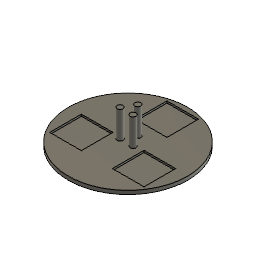
base (Autodesk Fusion 360 design; units mm, degrees)
Autodesk Fusion 360 part; units mm, degrees
note: some values were not read from the file. Set by a fixed rule: which sketch regions a step uses.
sketch "Sketch1" plane through (0, 0, 0) normal (0, 1, 0) x (1, 0, 0)
  line L0 (0, -25) -> (-12.5, -25)
  line L1 (-12.5, -25) -> (12.5, -25)
  line L2 (12.5, -25) -> (37.9, -25)
  circle A0 centre (0, 0) radius 48
  line L3 (37.9, -25) -> (12.5, -25)
  line L4 (12.5, -25) -> (12.5, 0.4)
  line L5 (12.5, 0.4) -> (37.9, 0.4)
  line L6 (37.9, 0.4) -> (37.9, -25)
  line L7 (-12.5, -25) -> (-37.9, -25)
  line L8 (-37.9, -25) -> (-37.9, 0.4)
  line L9 (-37.9, 0.4) -> (-12.5, 0.4)
  line L10 (-12.5, 0.4) -> (-12.5, -25)
  line L11 (-25.2, 0.4) -> (-25.2, -12.3)
  line L12 (12.5, 0.4) -> (25.2, 0.4)
  line L13 (25.2, 0.4) -> (25.2, -12.3)
  line L14 (-25.2, -12.3) -> (25.2, -12.3)
  line L15 (0, -12.3) -> (0, 31.347)
  line L16 (0, 31.347) -> (-25.2, -12.3)
  line L17 (25.2, -12.3) -> (0, 31.347)
  line L18 (0, 31.347) -> (0, 18.647)
  line L19 (0, 18.647) -> (12.7, 18.647)
  line L20 (12.7, 18.647) -> (-12.7, 18.647)
  line L21 (-12.7, 18.647) -> (-12.7, 44.047)
  line L22 (-12.7, 44.047) -> (12.7, 44.047)
  line L23 (12.7, 44.047) -> (12.7, 18.647)
  dimension "d2" = 12.5
  dimension "d3" = 25
  dimension "d4" = 25.4
  dimension "d5" = 96
  dimension "d6" = 25.4
  dimension "d7" = 25.4
  dimension "d8" = 25.4
  dimension "d9" = 25.4
  dimension "d10" = 12.7
  dimension "d11" = 12.7
  dimension "d12" = 12.7
  dimension "d13" = 43.647
  dimension "d14" = 12.7
  dimension "d15" = 12.7
  dimension "d16" = 25.4
  dimension "d17" = 25.4
  constraint horizontal L0
  constraint parallel L0 L1
  constraint parallel L1 L2
  constraint coincident A0.centre origin
  constraint horizontal L3
  constraint vertical L4
  constraint horizontal L5
  constraint vertical L6
  constraint horizontal L7
  constraint vertical L8
  constraint horizontal L9
  constraint vertical L10
  constraint midpoint L9 L11.start
  constraint perpendicular L9 L11
  constraint perpendicular L4 L12
  constraint perpendicular L12 L13
  constraint midpoint L14 L15.start
  constraint perpendicular L14 L15
  constraint parallel L15 L18
  constraint perpendicular L18 L19
  constraint horizontal L20
  constraint vertical L21
  constraint horizontal L22
  constraint vertical L23
  measures "d2" distance of L0.start L0.end
  measures "d3" distance of L0.end L1.end
  measures "d4" distance of L1.end L2.end
  measures "d5" diameter of A0
  measures "d6" distance of L2.end L1.end
  measures "d7" distance of L2.end L5.end
  measures "d8" distance of L0.end L7.end
  measures "d9" distance of L0.end L9.end
  measures "d10" distance of L11.start L11.end
  measures "d11" distance of L4.end L12.end
  measures "d12" distance of L12.end L13.end
  measures "d13" distance of L15.start L15.end
  measures "d14" distance of L15.end L18.end
  measures "d15" distance of L18.end L19.end
  measures "d16" distance of L19.end L20.end
  measures "d17" distance of L19.end L22.end
extrude "Extrude1" add sketch "Sketch1" along normal blind 3 contours L0 L1 L4 L10 L14 | L9 L10 L14 L15 L16 L20 | L4 L5 L12 L14 L15 L17 L19 L20 | A0
extrude "Extrude2" add sketch "Sketch1" along normal blind 1.5 contours L7 L8 L9 L10 L11 L14 | L2 L3 L4 L5 L6 L13 L14 | L9 L10 L14 L16 | L4 L5 L12 L14 L17 | L9 L11 L16 | L5 L12 L13 L17 | L15 L16 L18 L20 | L15 L17 L18 L19 L20 | L16 L17 L19 L20 L21 L22 L23
sketch "Sketch2" plane through (0, 3, 0) normal (0, 1, 0) x (-1, 0, 0)
  line L0 (-12.5, 25) -> (-12.5, -0.4)
  line L1 (-12.5, -0.4) -> (-37.9, -0.4)
  line L2 (-37.9, -0.4) -> (-37.9, 25)
  line L3 (-37.9, 25) -> (-12.5, 25)
  line L4 (12.7, -44.047) -> (-12.7, -44.047)
  line L5 (-12.7, -44.047) -> (-12.7, -18.647)
  line L6 (-12.7, -18.647) -> (12.7, -18.647)
  line L7 (12.7, -18.647) -> (12.7, -44.047)
  line L8 (37.9, -0.4) -> (12.5, -0.4)
  line L9 (12.5, -0.4) -> (12.5, 25)
  line L10 (12.5, 25) -> (37.9, 25)
  line L11 (37.9, 25) -> (37.9, -0.4)
  circle A0 centre (0, 0) radius 48
  line L12 (0, -31) -> (0, -1.902)
  circle A1 centre (0, -1.902) radius 10.5
  line L13 (0, -1.902) -> (0, -7.902)
  line L14 (0, -1.902) -> (-5.1962, 1.098)
  line L15 (0, -1.902) -> (5.1962, 1.098)
  line L16 (0, -1.902) -> (6, -1.902) construction
  circle A2 centre (0, -7.902) radius 2.35
  circle A3 centre (5.1962, 1.098) radius 2.35
  circle A4 centre (-5.1962, 1.098) radius 2.35
  dimension "d22" = 29.098
  dimension "d23" = 21
  dimension "d24" = 6
  dimension "d25" = 60
  dimension "d26" = 6
  dimension "d27" = 30
  dimension "d28" = 6
  dimension "d29" = 4.7
  dimension "d30" = 4.7
  dimension "d31" = 4.7
  constraint vertical L12
  constraint coincident L12.end A1.centre
  constraint parallel L12 L13
  constraint horizontal L16
  constraint coincident L13.end A2.centre
  constraint coincident L15.end A3.centre
  constraint coincident L14.end A4.centre
  measures "d22" distance of L12.start L12.end
  measures "d23" diameter of A1
  measures "d24" distance of L12.end L13.end
  measures "d25" angle of L13 L14
  measures "d26" distance of L12.end L14.end
  measures "d27" angle of L15 L16
  measures "d28" distance of L12.end L15.end
  measures "d29" diameter of A2
  measures "d30" diameter of A3
  measures "d31" diameter of A4
extrude "Extrude3" add sketch "Sketch2" along normal blind 22 contours L12 L13 A2 | L12 L13 A2 | A3 | A4
